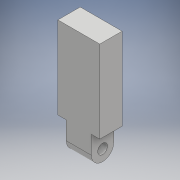
# Autodesk Inventor part: finger_long
Saved by Autodesk Inventor 2018 (Build 220112000, 112)
## iProperties
Created: 2018-04-12
Part Number: finger_long
Material: Genérico
Document SubType Name: Modeling
Designer: se_ma
Density: 1 g/cm^3
Appearance: Valor por defecto
Author: se_ma
Autodesk Inventor part; units mm, degrees
ref_plane "YZ Plane" through (0, 0, 0) normal (1, 0, 0) x (0, 1, 0)
ref_plane "XZ Plane" through (0, 0, 0) normal (0, 1, 0) x (-1, 0, 0)
ref_plane "XY Plane" through (0, 0, 0) normal (0, 0, 1) x (1, 0, 0)
sketch "Boceto1" plane through (0, 0, 0) normal (1, 0, 0) x (0, 1, 0)
  line L0 (0, 0) -> (-16, 0)
  line L1 (-16, 0) -> (-16, -70)
  line L2 (0, -70) -> (0, 0)
  line L3 (0, -70) -> (0, -80)
  line L4 (0, -80) -> (-16, -80)
  line L5 (-16, -80) -> (-16, -70)
  dimension "d0" = 16
  dimension "d1" = 70
  dimension "d2" = 10
  constraints: 12 end point, 3 perpendicular, 1 horizontal, 1 parallel, 1 vertical
  measures "d0" distance of L2.start L1.end
  measures "d1" distance of L1.end L0.end
  measures "d2" distance of L2.start L3.end
extrude "Extrusión1" add sketch "Boceto1" along normal blind 30
sketch "Boceto2" plane through (0, -16, -80) normal (0, 0, -1) x (-1, 0, 0)
  line L0 (0, 16) -> (-30, 16) projected
  line L1 (-15, 16) -> (-24, 16)
  line L2 (-24, 16) -> (-24, 0)
  line L3 (0, 0) -> (-30, 0) projected
  line L4 (-24, 0) -> (-30, 0)
  line L5 (-30, 16) -> (-30, 0) projected
  line L6 (-30, 0) -> (-30, 16)
  line L7 (-30, 16) -> (-24, 16)
  line L8 (-15, 16) -> (-6, 16)
  line L9 (-6, 16) -> (-6, 0)
  line L10 (0, 16) -> (0, 0) projected
  line L11 (-6, 0) -> (0, 0)
  line L12 (0, 0) -> (0, 16)
  line L13 (0, 16) -> (-6, 16)
  dimension "d5" = 9
  dimension "d6" = 9
  constraints: 20 end point, 7 perpendicular, 4 point on line, 1 horizontal, 1 midpoint
  measures "d5" distance of L1.start L1.end
  measures "d6" distance of L1.start L8.end
extrude "Extrusión2" cut sketch "Boceto2" against normal blind 21 contours L10 L3 L9 L0 | L2 L3 L5 L0
sketch "Boceto3" plane through (24, -16, -80) normal (1, 0, 0) x (0, 0, -1)
  line L0 (-21, 16) -> (0, 16) projected
  line L1 (0, 16) -> (-8, 16)
  line L2 (-8, 16) -> (-8, 0)
  line L3 (0, 0) -> (-21, 0) projected
  arc A0 (-8, 0) -> (-8, 16) centre (-8, 8) ccw
  circle A1 centre (-8, 8) radius 3.5
  line L4 (0, 16) -> (0, 8)
  line L5 (0, 16) -> (0, 0) projected
  line L6 (0, 8) -> (0, 0)
  line L7 (0, 0) -> (-8, 0)
  point P0 (-80, 16)
  dimension "d9" = 8
  dimension "d10" = 7
  constraints: 10 end point, 2 centre point, 2 midpoint, 2 point on circle, 2 point on line, 1 coincident, 1 collinear, 1 perpendicular
  measures "d9" distance of L0.end L1.end
  measures "d10" diameter of A1
extrude "Extrusión3" cut sketch "Boceto3" against normal blind 18 contours L0 L4 A0 | A1 L2 | L2 A1 | L5 L3 A0
